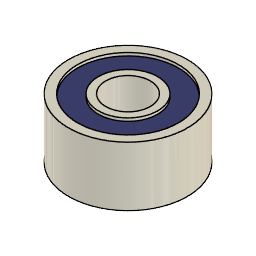
Bearing_v1 (Autodesk Fusion 360 design; units mm, degrees)
Autodesk Fusion 360 part; units mm, degrees
sketch "Sketch1" plane through (0, 0, 0) normal (0, 0, 1) x (1, 0, 0)
  circle A0 centre (0, 0) radius 1.5
  circle A1 centre (0, 0) radius 4
  circle A2 centre (0, 0) radius 3.4
  circle A3 centre (0, 0) radius 2
  dimension "d1" = 3
  dimension "d2" = 8
  dimension "d3" = -0.6
  dimension "d4" = 0.5
  constraint coincident A0.centre A1.centre
  measures "d1" diameter of A0
  measures "d2" diameter of A1
extrude "Extrude1" add sketch "Sketch1" along normal mid plane 4 makes body 1 at (3.995, -0.1994, 1.3333) makes body 2 at (1.9975, -0.0997, 1.3333)
extrude "Extrude2" add sketch "Sketch1" along normal mid plane 3.6 contours A2 bodies 1 2
